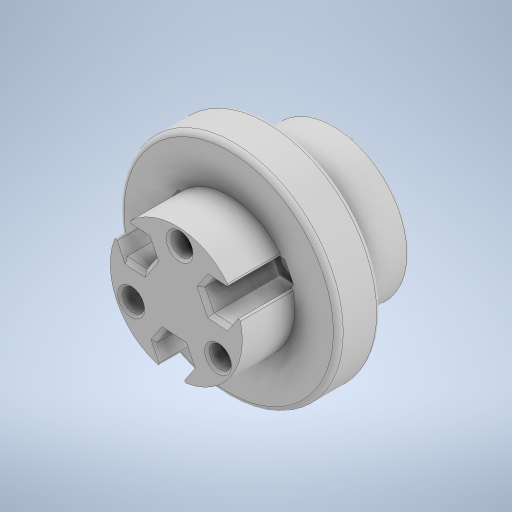
# Autodesk Inventor part: Os_lewa
Saved by Autodesk Inventor 2023 (Build 270158000, 158)
## iProperties
Created: 2023-01-20
Part Number: Os_lewa
Material: Generic
Document SubType Name: Modeling
Designer: Kamil
Density: 1 g/cm^3
Appearance: Default
Mass: 24.6075 g
Surface Area: 89.1781 cm^2
Volume: 24.6075 cm^3
Author: Kamil
Autodesk Inventor part; units mm, degrees
ref_plane "YZ Plane" through (0, 0, 0) normal (1, 0, 0) x (0, 1, 0)
ref_plane "XZ Plane" through (0, 0, 0) normal (0, 1, 0) x (-1, 0, 0)
sketch "Sketch1" plane through (0, 0, 0) normal (0, 0, 1) x (1, 0, 0)
  circle A0 centre (0, 0) radius 23.3333 projected
  arc A1 (-39.2843, 4.1223) -> (-36.4252, -2.8784) centre (-31.328, 3.2874) ccw projected
  arc A2 (-35.6202, -8.1415) -> (-36.4252, -2.8784) centre (-38.9739, -5.9614) ccw projected
  arc A3 (-35.6202, -8.1415) -> (-36.2558, -15.6768) centre (-28.9129, -12.5018) ccw projected
  arc A4 (-36.2558, -15.6768) -> (33.8969, -20.2792) centre (0, 0) ccw projected
  arc A5 (33.8969, -20.2792) -> (34.2512, -12.7254) centre (27.0317, -16.172) ccw projected
  arc A6 (35.737, -7.6127) -> (34.2512, -12.7254) centre (37.861, -11.0021) ccw projected
  arc A7 (35.737, -7.6127) -> (39.4862, -1.0454) centre (31.489, -0.8337) ccw projected
  arc A8 (39.4862, -1.0454) -> (-39.2843, 4.1223) centre (0, 0) ccw projected
  circle A9 centre (-9.1932, -4.5329) radius 2 projected
  circle A10 centre (9.1932, 4.5329) radius 2 projected
  circle A11 centre (-0.671, -10.228) radius 2 projected
  circle A12 centre (-8.5222, 5.6951) radius 2 projected
  circle A13 centre (0.671, 10.228) radius 2 projected
  circle A14 centre (8.5222, -5.6951) radius 2 projected
  circle A15 centre (0, 0) radius 13.4591 projected
  line L0 (-5.9382, 0.859) -> (-7.1311, 0.7284) projected
  arc A16 (-5.6118, -2.1232) -> (-5.9382, 0.859) centre (0, 0) ccw projected
  line L1 (-6.8047, -2.2538) -> (-5.6118, -2.1232) projected
  line L2 (-7.1311, 0.7284) -> (-6.8047, -2.2538) projected
  line L3 (23.3333, 0) -> (22.3333, 0)
  circle A17 centre (0, 0) radius 22.3333
  circle A18 centre (0, 0) radius 6
  circle A19 centre (16.7628, -26.571) radius 3.75 projected
  circle A20 centre (-29.1794, 11.6435) radius 3.75 projected
  circle A21 centre (2.0567, 31.3493) radius 3.75 projected
  circle A22 centre (-20.0905, -24.1532) radius 3.75 projected
  circle A23 centre (30.4505, 7.7314) radius 3.75 projected
  point P0 (0, 0)
  dimension "d0" = 1
  constraints: 2 coincident, 2 end point, 2 horizontal alignment, 1 horizontal, 6 other
  measures "d0" distance of L3.start L3.end
extrude "Extrusion1" add sketch "Sketch1" along normal blind 3.8 contours A15 | A18 L1 L2 L0 | A16 A18 | A17
sketch "Sketch2" plane through (0, 0, 0) normal (0, 0, -1) x (-1, 0, 0)
  circle A0 centre (0, 0) radius 15 projected
  circle A1 centre (0, 0) radius 22.3333 projected
  circle A2 centre (9.1932, -4.5329) radius 2 projected
  circle A3 centre (-9.1932, 4.5329) radius 2 projected
  circle A4 centre (0.671, -10.228) radius 2 projected
  circle A5 centre (8.5222, 5.6951) radius 2 projected
  circle A6 centre (-0.671, 10.228) radius 2 projected
  circle A7 centre (-8.5222, -5.6951) radius 2 projected
  point P0 (0, 0)
ref_plane "Work Plane1" through (-21.6708, -21.6708, -13) normal (0, 0, -1) x (0, 1, 0)
extrude "Extrusion2" add sketch "Sketch2" along normal up to surface (13 mm away) contours A0
sketch "Sketch3" plane through (0, 0, 3.8) normal (0, 0, 1) x (1, 0, 0)
  point P0 (0, 0)
sketch "Sketch4" plane through (0, 0, -13) normal (0, 0, -1) x (-1, 0, 0)
  circle A0 centre (0, 0) radius 15 projected
  circle A1 centre (-8.5222, -5.6951) radius 2 projected
  circle A2 centre (-0.671, 10.228) radius 2 projected
  circle A3 centre (8.5222, 5.6951) radius 2 projected
  circle A4 centre (0.671, -10.228) radius 2 projected
  circle A5 centre (-9.1932, 4.5329) radius 2 projected
  circle A6 centre (9.1932, -4.5329) radius 2 projected
  line L0 (0, 0) -> (9.1932, -4.5329)
  line L1 (9.1932, -4.5329) -> (12.3324, -6.0807)
  circle A7 centre (9.1932, -4.5329) radius 2 projected
  circle A8 centre (9.1932, -4.5329) radius 3.5
  circle A9 centre (8.5222, 5.6951) radius 3.5
  circle A10 centre (-0.671, 10.228) radius 3.5
  circle A11 centre (-9.1932, 4.5329) radius 3.5
  circle A12 centre (-8.5222, -5.6951) radius 3.5
  circle A13 centre (0.671, -10.228) radius 3.5
  point P0 (0, 0)
  point P1 (11.4322, 7.6398)
  point P2 (-0.9001, 13.7205)
  point P3 (-12.3324, 6.0807)
  point P4 (-11.4322, -7.6398)
  point P5 (0.9001, -13.7205)
  dimension "d5" = 3.5
  dimension "d8" = 360
  constraints: 4 end point, 1 coincident, 1 collinear, 37 other
  measures "d5" distance of L0.end L1.end
extrude "Extrusion3" cut sketch "Sketch4" against normal blind 5 contours A1 | A6 L1 L0 | A6 L0 A8 L1 | L0 L1 A6 | A6 L1 A8 L0 | A10 | A12
sketch "Sketch5" plane through (0, 0, 3.8) normal (0, 0, 1) x (1, 0, 0)
  circle A0 centre (0, 0) radius 22.3333 projected
  circle A1 centre (-9.1932, -4.5329) radius 2 projected
  circle A2 centre (9.1932, 4.5329) radius 2 projected
  circle A3 centre (-0.671, -10.228) radius 2 projected
  circle A4 centre (-8.5222, 5.6951) radius 2 projected
  circle A5 centre (0.671, 10.228) radius 2 projected
  circle A6 centre (8.5222, -5.6951) radius 2 projected
  line L0 (0, 0) -> (-0.671, -10.228)
  circle A7 centre (-0.671, -10.228) radius 2 projected
  line L1 (-0.671, -10.228) -> (-1.462, -22.2854)
  circle A8 centre (0, 0) radius 22.3333 projected
  line L2 (-0.671, -10.228) -> (-0.9001, -13.7205)
  line L3 (-3.0871, -13.8731) -> (-5.0083, -9.9765)
  line L4 (-5.0083, -9.9765) -> (-2.5944, -6.3644)
  line L5 (-2.5944, -6.3644) -> (1.7407, -6.6488)
  line L6 (1.7407, -6.6488) -> (3.662, -10.5454)
  line L7 (3.662, -10.5454) -> (1.2481, -14.1575)
  line L8 (1.2481, -14.1575) -> (-3.0871, -13.8731)
  line L9 (4.2145, -5.429) -> (6.6284, -1.8169)
  line L10 (6.1358, -9.3256) -> (4.2145, -5.429)
  line L11 (10.4709, -9.61) -> (6.1358, -9.3256)
  line L12 (12.8848, -5.9979) -> (10.4709, -9.61)
  line L13 (10.9635, -2.1013) -> (12.8848, -5.9979)
  line L14 (6.6284, -1.8169) -> (10.9635, -2.1013)
  line L15 (6.8089, 0.9353) -> (4.8877, 4.8319)
  line L16 (11.1441, 0.6509) -> (6.8089, 0.9353)
  line L17 (13.558, 4.2631) -> (11.1441, 0.6509)
  line L18 (11.6367, 8.1596) -> (13.558, 4.2631)
  line L19 (7.3016, 8.4441) -> (11.6367, 8.1596)
  line L20 (4.8877, 4.8319) -> (7.3016, 8.4441)
  line L21 (2.5944, 6.3644) -> (-1.7407, 6.6488)
  line L22 (5.0083, 9.9765) -> (2.5944, 6.3644)
  line L23 (3.0871, 13.8731) -> (5.0083, 9.9765)
  line L24 (-1.2481, 14.1575) -> (3.0871, 13.8731)
  line L25 (-3.662, 10.5454) -> (-1.2481, 14.1575)
  line L26 (-1.7407, 6.6488) -> (-3.662, 10.5454)
  line L27 (-4.2145, 5.429) -> (-6.6284, 1.8169)
  line L28 (-6.1358, 9.3256) -> (-4.2145, 5.429)
  line L29 (-10.4709, 9.61) -> (-6.1358, 9.3256)
  line L30 (-12.8848, 5.9979) -> (-10.4709, 9.61)
  line L31 (-10.9635, 2.1013) -> (-12.8848, 5.9979)
  line L32 (-6.6284, 1.8169) -> (-10.9635, 2.1013)
  line L33 (-6.8089, -0.9353) -> (-4.8877, -4.8319)
  line L34 (-11.1441, -0.6509) -> (-6.8089, -0.9353)
  line L35 (-13.558, -4.2631) -> (-11.1441, -0.6509)
  line L36 (-11.6367, -8.1596) -> (-13.558, -4.2631)
  line L37 (-7.3016, -8.4441) -> (-11.6367, -8.1596)
  line L38 (-4.8877, -4.8319) -> (-7.3016, -8.4441)
  point P0 (0, 0)
  point P1 (-0.6732, -10.261)
  point P2 (-0.9195, -14.0153)
  point P3 (11.6779, -7.8039)
  point P4 (12.5974, 6.2114)
  point P5 (0.9195, 14.0153)
  point P6 (-11.6779, 7.8039)
  point P7 (-12.5974, -6.2114)
  dimension "d13" = 3.5
  dimension "d16" = 360
  constraints: 78 end point, 2 point on line, 1 collinear, 1 midpoint, 94 other
  measures "d13" distance of L1.start L2.end
extrude "Extrusion4" add sketch "Sketch5" along normal blind 5 contours A0 | L9 L14 L13 L12 L11 L10 | L21 L26 L25 L24 L23 L22 | L33 L38 L37 L36 L35 L34
sketch "Sketch6" plane through (0, 0, 3.8) normal (0, 0, 1) x (1, 0, 0)
  line L0 (6.8089, 0.9353) -> (11.1441, 0.6509) projected
  line L1 (11.1441, 0.6509) -> (13.558, 4.2631) projected
  line L2 (13.558, 4.2631) -> (11.6367, 8.1596) projected
  line L3 (11.6367, 8.1596) -> (7.3016, 8.4441) projected
  line L4 (7.3016, 8.4441) -> (4.8877, 4.8319) projected
  line L5 (4.8877, 4.8319) -> (6.8089, 0.9353) projected
  circle A0 centre (9.1932, 4.5329) radius 2 projected
  circle A1 centre (0, 0) radius 22.3333 projected
  circle A2 centre (8.5222, -5.6951) radius 2 projected
  circle A3 centre (0.671, 10.228) radius 2 projected
  circle A4 centre (-9.1932, -4.5329) radius 2 projected
  line L6 (1.2481, -14.1575) -> (-3.0871, -13.8731) projected
  line L7 (-3.0871, -13.8731) -> (-5.0083, -9.9765) projected
  line L8 (-5.0083, -9.9765) -> (-2.5944, -6.3644) projected
  line L9 (-2.5944, -6.3644) -> (1.7407, -6.6488) projected
  line L10 (1.7407, -6.6488) -> (3.662, -10.5454) projected
  line L11 (3.662, -10.5454) -> (1.2481, -14.1575) projected
  line L12 (-4.2145, 5.429) -> (-6.6284, 1.8169) projected
  line L13 (-6.6284, 1.8169) -> (-10.9635, 2.1013) projected
  line L14 (-10.9635, 2.1013) -> (-12.8848, 5.9979) projected
  line L15 (-12.8848, 5.9979) -> (-10.4709, 9.61) projected
  line L16 (-10.4709, 9.61) -> (-6.1358, 9.3256) projected
  line L17 (-6.1358, 9.3256) -> (-4.2145, 5.429) projected
  line L18 (6.8089, 0.9353) -> (4.8877, 4.8319) projected
  line L19 (4.8877, 4.8319) -> (7.3016, 8.4441) projected
  line L20 (7.3016, 8.4441) -> (11.6367, 8.1596) projected
  line L21 (11.6367, 8.1596) -> (13.558, 4.2631) projected
  line L22 (13.558, 4.2631) -> (11.1441, 0.6509) projected
  line L23 (11.1441, 0.6509) -> (6.8089, 0.9353) projected
  circle A5 centre (-0.671, -10.228) radius 2 projected
  circle A6 centre (-8.5222, 5.6951) radius 2 projected
  point P0 (0, 0)
extrude "Extrusion5" add sketch "Sketch6" along normal blind 1.5 contours L5 L4 L3 L2 L1 L0 | L6 L7 L8 L9 L10 L11 | L12 L13 L14 L15 L16 L17
sketch "Sketch7" plane through (0, 0, 8.8) normal (0, 0, 1) x (1, 0, 0)
  circle A0 centre (8.5222, -5.6951) radius 2 projected
  circle A1 centre (9.1932, 4.5329) radius 2 projected
  circle A2 centre (-0.671, -10.228) radius 2 projected
  circle A3 centre (0.671, 10.228) radius 2 projected
  circle A4 centre (-9.1932, -4.5329) radius 2 projected
  arc A5 (5.9995, 0.0758) -> (5.2863, -2.8382) centre (0, 0) ccw projected
  line L0 (7.1651, -0.2095) -> (5.9995, 0.0758) projected
  line L1 (6.4519, -3.1235) -> (7.1651, -0.2095) projected
  line L2 (5.2863, -2.8382) -> (6.4519, -3.1235) projected
  circle A6 centre (-8.5222, 5.6951) radius 2 projected
  circle A7 centre (0, 0) radius 13.4542 projected
  circle A8 centre (0, 0) radius 6
  circle A9 centre (0, 0) radius 22.3333 projected
  circle A10 centre (8.5222, -5.6951) radius 2 projected
  circle A11 centre (0.671, 10.228) radius 2 projected
  circle A12 centre (-9.1932, -4.5329) radius 2 projected
  line L3 (1.2481, -14.1575) -> (-3.0871, -13.8731) projected
  line L4 (-3.0871, -13.8731) -> (-5.0083, -9.9765) projected
  line L5 (-5.0083, -9.9765) -> (-2.5944, -6.3644) projected
  line L6 (-2.5944, -6.3644) -> (1.7407, -6.6488) projected
  line L7 (1.7407, -6.6488) -> (3.662, -10.5454) projected
  line L8 (3.662, -10.5454) -> (1.2481, -14.1575) projected
  line L9 (-4.2145, 5.429) -> (-6.6284, 1.8169) projected
  line L10 (-6.6284, 1.8169) -> (-10.9635, 2.1013) projected
  line L11 (-10.9635, 2.1013) -> (-12.8848, 5.9979) projected
  line L12 (-12.8848, 5.9979) -> (-10.4709, 9.61) projected
  line L13 (-10.4709, 9.61) -> (-6.1358, 9.3256) projected
  line L14 (-6.1358, 9.3256) -> (-4.2145, 5.429) projected
  line L15 (6.8089, 0.9353) -> (4.8877, 4.8319) projected
  line L16 (4.8877, 4.8319) -> (7.3016, 8.4441) projected
  line L17 (7.3016, 8.4441) -> (11.6367, 8.1596) projected
  line L18 (11.6367, 8.1596) -> (13.558, 4.2631) projected
  line L19 (13.558, 4.2631) -> (11.1441, 0.6509) projected
  line L20 (11.1441, 0.6509) -> (6.8089, 0.9353) projected
  point P0 (0, 0)
  point P1 (1.7989, -13.3334)
  point P2 (13.0072, 3.4389)
  point P3 (10.6476, 8.2245)
  point P4 (-9.4818, 9.5451)
  point P5 (-12.4465, 5.1088)
  point P6 (-3.5254, -12.9841)
  constraints: 1 coincident, 3 other
extrude "Extrusion6" add sketch "Sketch7" along normal blind 5.2 contours L0 L1 L2 A8 | A7 L8 L7 L6 L5 L4 L11 L10 L9 L14 L13 L17 L16 L15 L20 L19
sketch "Sketch8" plane through (-9.1932, -4.5329, -8) normal (0, 0, -1) x (-1, 0, 0)
  circle A0 centre (0, 0) radius 2 projected
  circle A1 centre (0, 0) radius 3.5 projected
  circle A2 centre (-9.8642, 14.7609) radius 3.5 projected
  circle A3 centre (-17.7154, -1.1622) radius 3.5 projected
  circle A4 centre (0, 0) radius 3.5 projected
  circle A5 centre (-9.1932, 4.5329) radius 15 projected
  circle A6 centre (-0.671, 10.228) radius 2 projected
  circle A7 centre (-8.5222, -5.6951) radius 2 projected
  circle A8 centre (-18.3864, 9.0658) radius 2 projected
  line L0 (0, 0) -> (-18.3864, 9.0658)
  line L1 (-17.7154, -1.1622) -> (-0.671, 10.228)
  line L2 (-8.5222, -5.6951) -> (-9.8642, 14.7609)
  line L3 (0, 0) -> (3.1391, -1.5478)
  line L4 (2.2455, -3.3602) -> (-1.7873, -3.6248)
  line L5 (-1.7873, -3.6248) -> (-4.0328, -0.2646)
  line L6 (-4.0328, -0.2646) -> (-2.2455, 3.3602)
  line L7 (-2.2455, 3.3602) -> (1.7873, 3.6248)
  line L8 (1.7873, 3.6248) -> (4.0328, 0.2646)
  line L9 (4.0328, 0.2646) -> (2.2455, -3.3602)
  line L10 (3.3618, 10.4926) -> (1.5745, 6.8678)
  line L11 (1.5745, 6.8678) -> (-2.4583, 6.6032)
  line L12 (-2.4583, 6.6032) -> (-4.7038, 9.9634)
  line L13 (-4.7038, 9.9634) -> (-2.9165, 13.5882)
  line L14 (-2.9165, 13.5882) -> (1.1163, 13.8528)
  line L15 (1.1163, 13.8528) -> (3.3618, 10.4926)
  line L16 (-8.077, 18.3857) -> (-5.8315, 15.0255)
  line L17 (-5.8315, 15.0255) -> (-7.6187, 11.4007)
  line L18 (-7.6187, 11.4007) -> (-11.6515, 11.1361)
  line L19 (-11.6515, 11.1361) -> (-13.897, 14.4963)
  line L20 (-13.897, 14.4963) -> (-12.1097, 18.1211)
  line L21 (-12.1097, 18.1211) -> (-8.077, 18.3857)
  line L22 (-20.632, 12.426) -> (-16.5992, 12.6906)
  line L23 (-16.5992, 12.6906) -> (-14.3537, 9.3304)
  line L24 (-14.3537, 9.3304) -> (-16.1409, 5.7056)
  line L25 (-16.1409, 5.7056) -> (-20.1737, 5.441)
  line L26 (-20.1737, 5.441) -> (-22.4192, 8.8012)
  line L27 (-22.4192, 8.8012) -> (-20.632, 12.426)
  line L28 (-21.7482, -1.4268) -> (-19.961, 2.198)
  line L29 (-19.961, 2.198) -> (-15.9282, 2.4626)
  line L30 (-15.9282, 2.4626) -> (-13.6827, -0.8977)
  line L31 (-13.6827, -0.8977) -> (-15.4699, -4.5224)
  line L32 (-15.4699, -4.5224) -> (-19.5027, -4.787)
  line L33 (-19.5027, -4.787) -> (-21.7482, -1.4268)
  line L34 (-10.3095, -9.3199) -> (-12.555, -5.9597)
  line L35 (-12.555, -5.9597) -> (-10.7677, -2.3349)
  line L36 (-10.7677, -2.3349) -> (-6.7349, -2.0703)
  line L37 (-6.7349, -2.0703) -> (-4.4894, -5.4305)
  line L38 (-4.4894, -5.4305) -> (-6.2767, -9.0553)
  line L39 (-6.2767, -9.0553) -> (-10.3095, -9.3199)
  point P0 (-9.1932, 4.5329)
  point P1 (2.239, 12.1727)
  point P2 (-10.0934, 18.2534)
  point P3 (-21.5256, 10.6136)
  point P4 (-20.6255, -3.1069)
  point P5 (-8.2931, -9.1876)
  dimension "d24" = 3.5
  dimension "d27" = 360
  constraints: 80 end point, 1 coincident, 1 collinear, 1 midpoint, 92 other
  measures "d24" distance of L0.start L3.end
extrude "Extrusion7" cut sketch "Sketch8" along normal blind 10 contours A0 L3 L0 | A0 L0 A1 L3 | L0 L3 A0 | A0 L3 A1 L0 | L6 L7 A1 | A1 L5 L6 | L9 L4 A1 | A1 L8 L9 | L7 L8 A1 | A1 L4 L5 | A2 | A2 L16 L17 | A2 L21 L16 | L17 L18 A2 | A2 L20 L21 | L18 L19 A2 | A2 L19 L20 | A3 | A3 L30 L31 | A3 L29 L30 | L31 L32 A3 | A3 L28 L29 | L32 L33 A3 | A3 L33 L28
sketch "Sketch9" plane through (0, 0, 8.8) normal (0, 0, 1) x (1, 0, 0)
  circle A0 centre (0, 0) radius 6 projected
  point P0 (0, 0)
extrude "Extrusion8" add sketch "Sketch9" along normal up to surface (5.2 mm away)
sketch "Sketch10" plane through (0, 0, 14) normal (0, 0, 1) x (1, 0, 0)
  line L0 (3.662, -10.5454) -> (1.7989, -13.3334) projected
  arc A0 (1.7989, -13.3334) -> (13.0072, 3.4389) centre (0, 0) ccw projected
  line L1 (13.0072, 3.4389) -> (11.1441, 0.6509) projected
  line L2 (11.1441, 0.6509) -> (6.8089, 0.9353) projected
  line L3 (6.8089, 0.9353) -> (4.8877, 4.8319) projected
  line L4 (4.8877, 4.8319) -> (7.3016, 8.4441) projected
  line L5 (7.3016, 8.4441) -> (10.6476, 8.2245) projected
  arc A1 (10.6476, 8.2245) -> (-9.4818, 9.5451) centre (0, 0) ccw projected
  line L6 (-9.4818, 9.5451) -> (-6.1358, 9.3256) projected
  line L7 (-6.1358, 9.3256) -> (-4.2145, 5.429) projected
  line L8 (-4.2145, 5.429) -> (-6.6284, 1.8169) projected
  line L9 (-6.6284, 1.8169) -> (-10.9635, 2.1013) projected
  line L10 (-10.9635, 2.1013) -> (-12.4465, 5.1088) projected
  arc A2 (-12.4465, 5.1088) -> (-3.5254, -12.9841) centre (0, 0) ccw projected
  line L11 (-3.5254, -12.9841) -> (-5.0083, -9.9765) projected
  line L12 (-5.0083, -9.9765) -> (-2.5944, -6.3644) projected
  line L13 (-2.5944, -6.3644) -> (1.7407, -6.6488) projected
  line L14 (1.7407, -6.6488) -> (3.662, -10.5454) projected
  circle A3 centre (8.5222, -5.6951) radius 2 projected
  circle A4 centre (0.671, 10.228) radius 2 projected
  circle A5 centre (-9.1932, -4.5329) radius 2 projected
  point P0 (0, 0)
extrude "Extrusion9" add sketch "Sketch10" along normal blind 5.5
sketch "Sketch11" plane through (0, 0, 19.5) normal (0, 0, 1) x (1, 0, 0)
  line L0 (-5.0083, -9.9765) -> (-2.5944, -6.3644) projected
  line L1 (-2.5944, -6.3644) -> (1.7407, -6.6488) projected
  line L2 (1.7407, -6.6488) -> (3.662, -10.5454) projected
  line L3 (11.1441, 0.6509) -> (6.8089, 0.9353) projected
  line L4 (6.8089, 0.9353) -> (4.8877, 4.8319) projected
  line L5 (4.8877, 4.8319) -> (7.3016, 8.4441) projected
  line L6 (-6.1358, 9.3256) -> (-4.2145, 5.429) projected
  line L7 (-4.2145, 5.429) -> (-6.6284, 1.8169) projected
  line L8 (-6.6284, 1.8169) -> (-10.9635, 2.1013) projected
  circle A0 centre (-9.1932, -4.5329) radius 2 projected
  circle A1 centre (0.671, 10.228) radius 2 projected
  circle A2 centre (8.5222, -5.6951) radius 2 projected
  circle A3 centre (-8.5222, 5.6951) radius 2 projected
  circle A4 centre (-0.671, -10.228) radius 2 projected
  circle A5 centre (9.1932, 4.5329) radius 2 projected
  circle A6 centre (-8.5222, 5.6951) radius 2 projected
  circle A7 centre (-8.5222, 5.6951) radius 2.25
  circle A8 centre (0.671, 10.228) radius 2 projected
  circle A9 centre (0.671, 10.228) radius 2.25
  circle A10 centre (9.1932, 4.5329) radius 2.25
  circle A11 centre (-0.671, -10.228) radius 2 projected
  circle A12 centre (-0.671, -10.228) radius 2.25
  circle A13 centre (-9.1932, -4.5329) radius 2.25
  circle A14 centre (8.5222, -5.6951) radius 2.25
  line L9 (-3.5254, -12.9841) -> (-5.0083, -9.9765) projected
  line L10 (3.662, -10.5454) -> (1.7989, -13.3334) projected
  line L11 (13.0072, 3.4389) -> (11.1441, 0.6509) projected
  line L12 (7.3016, 8.4441) -> (10.6476, 8.2245) projected
  line L13 (-9.4818, 9.5451) -> (-6.1358, 9.3256) projected
  line L14 (-10.9635, 2.1013) -> (-12.4465, 5.1088) projected
  arc A15 (1.7989, -13.3334) -> (13.0072, 3.4389) centre (0, 0) ccw projected
  arc A16 (10.6476, 8.2245) -> (-9.4818, 9.5451) centre (0, 0) ccw projected
  arc A17 (-12.4465, 5.1088) -> (-3.5254, -12.9841) centre (0, 0) ccw projected
  point P0 (0, 0)
  dimension "d37" = 4.5
  dimension "d38" = 4.5
  dimension "d39" = 4.5
  dimension "d40" = 4.5
  dimension "d41" = 4.5
  dimension "d42" = 4.5
  constraints: 6 centre point, 6 coincident
  measures "d37" diameter of A7
  measures "d38" diameter of A9
  measures "d39" diameter of A10
  measures "d40" diameter of A12
  measures "d41" diameter of A13
  measures "d42" diameter of A14
extrude "Extrusion10" cut sketch "Sketch11" against normal through all contours A0 | A1 | A2 | A3 | A4 | A5 | A7 | A9 | A10 | A12 | A13 | A14
sketch "Sketch13" plane through (0, 0, -8) normal (0, 0, -1) x (-1, 0, 0)
  circle A0 centre (-8.5222, -5.6951) radius 2.25 projected
  line L0 (-6.7349, -2.0703) -> (-10.7677, -2.3349) projected
  line L1 (-10.7677, -2.3349) -> (-12.555, -5.9597) projected
  line L2 (-12.555, -5.9597) -> (-10.3095, -9.3199) projected
  line L3 (-10.3095, -9.3199) -> (-6.2767, -9.0553) projected
  line L4 (-6.2767, -9.0553) -> (-4.4894, -5.4305) projected
  line L5 (-4.4894, -5.4305) -> (-6.7349, -2.0703) projected
  circle A1 centre (9.1932, -4.5329) radius 2.25 projected
  line L6 (13.226, -4.2683) -> (10.9805, -0.9081) projected
  line L7 (10.9805, -0.9081) -> (6.9477, -1.1727) projected
  line L8 (6.9477, -1.1727) -> (5.1604, -4.7975) projected
  line L9 (5.1604, -4.7975) -> (7.406, -8.1577) projected
  line L10 (7.406, -8.1577) -> (11.4387, -7.8931) projected
  line L11 (11.4387, -7.8931) -> (13.226, -4.2683) projected
  circle A2 centre (-0.671, 10.228) radius 2.25 projected
  line L12 (1.5745, 6.8678) -> (3.3618, 10.4926) projected
  line L13 (3.3618, 10.4926) -> (1.1163, 13.8528) projected
  line L14 (1.1163, 13.8528) -> (-2.9165, 13.5882) projected
  line L15 (-2.9165, 13.5882) -> (-4.7038, 9.9634) projected
  line L16 (-4.7038, 9.9634) -> (-2.4583, 6.6032) projected
  line L17 (-2.4583, 6.6032) -> (1.5745, 6.8678) projected
  point P0 (0, 0)
extrude "Extrusion12" cut sketch "Sketch13" against normal blind 3
sketch "Szkic14" plane through (0, 0, 5.3) normal (0, 0, 1) x (1, 0, 0)
  circle A0 centre (-8.5222, 5.6951) radius 2.25 projected
  line L0 (-10.4709, 9.61) -> (-6.1358, 9.3256) projected
  line L1 (-12.8848, 5.9979) -> (-10.4709, 9.61) projected
  line L2 (-10.9635, 2.1013) -> (-12.8848, 5.9979) projected
  line L3 (-6.6284, 1.8169) -> (-10.9635, 2.1013) projected
  line L4 (-4.2145, 5.429) -> (-6.6284, 1.8169) projected
  line L5 (-6.1358, 9.3256) -> (-4.2145, 5.429) projected
  circle A1 centre (-0.671, -10.228) radius 2.25 projected
  line L6 (1.7407, -6.6488) -> (3.662, -10.5454) projected
  line L7 (-2.5944, -6.3644) -> (1.7407, -6.6488) projected
  line L8 (-5.0083, -9.9765) -> (-2.5944, -6.3644) projected
  line L9 (-3.0871, -13.8731) -> (-5.0083, -9.9765) projected
  line L10 (1.2481, -14.1575) -> (-3.0871, -13.8731) projected
  line L11 (3.662, -10.5454) -> (1.2481, -14.1575) projected
  circle A2 centre (9.1932, 4.5329) radius 2.25 projected
  line L12 (11.1441, 0.6509) -> (6.8089, 0.9353) projected
  line L13 (13.558, 4.2631) -> (11.1441, 0.6509) projected
  line L14 (11.6367, 8.1596) -> (13.558, 4.2631) projected
  line L15 (7.3016, 8.4441) -> (11.6367, 8.1596) projected
  line L16 (4.8877, 4.8319) -> (7.3016, 8.4441) projected
  line L17 (6.8089, 0.9353) -> (4.8877, 4.8319) projected
  line L18 (-8.5222, 5.6951) -> (-8.2931, 9.1876)
  line L19 (-6.2767, 9.0553) -> (-4.4894, 5.4305)
  line L20 (-4.4894, 5.4305) -> (-6.7349, 2.0703)
  line L21 (-6.7349, 2.0703) -> (-10.7677, 2.3349)
  line L22 (-10.7677, 2.3349) -> (-12.555, 5.9597)
  line L23 (-12.555, 5.9597) -> (-10.3095, 9.3199)
  line L24 (-10.3095, 9.3199) -> (-6.2767, 9.0553)
  line L25 (-9.4818, 9.5451) -> (-6.1358, 9.3256) projected
  circle A3 centre (-9.1932, -4.5329) radius 2.25 projected
  circle A4 centre (0.671, 10.228) radius 2.25 projected
  circle A5 centre (8.5222, -5.6951) radius 2.25 projected
  arc A6 (1.7989, -13.3334) -> (13.0072, 3.4389) centre (0, 0) ccw projected
  line L26 (13.0072, 3.4389) -> (11.1441, 0.6509) projected
  line L27 (11.1441, 0.6509) -> (6.8089, 0.9353) projected
  line L28 (6.8089, 0.9353) -> (4.8877, 4.8319) projected
  line L29 (4.8877, 4.8319) -> (7.3016, 8.4441) projected
  line L30 (7.3016, 8.4441) -> (10.6476, 8.2245) projected
  arc A7 (10.6476, 8.2245) -> (-9.4818, 9.5451) centre (0, 0) ccw projected
  line L31 (-9.4818, 9.5451) -> (-6.1358, 9.3256) projected
  line L32 (-6.1358, 9.3256) -> (-4.2145, 5.429) projected
  line L33 (-4.2145, 5.429) -> (-6.6284, 1.8169) projected
  line L34 (-6.6284, 1.8169) -> (-10.9635, 2.1013) projected
  line L35 (-10.9635, 2.1013) -> (-12.4465, 5.1088) projected
  arc A8 (-12.4465, 5.1088) -> (-3.5254, -12.9841) centre (0, 0) ccw projected
  line L36 (-3.5254, -12.9841) -> (-5.0083, -9.9765) projected
  line L37 (-5.0083, -9.9765) -> (-2.5944, -6.3644) projected
  line L38 (-2.5944, -6.3644) -> (1.7407, -6.6488) projected
  line L39 (1.7407, -6.6488) -> (3.662, -10.5454) projected
  line L40 (3.662, -10.5454) -> (1.7989, -13.3334) projected
  arc A9 (10.6476, 8.2245) -> (-9.4818, 9.5451) centre (0, 0) ccw projected
  line L41 (10.6476, 8.2245) -> (11.6367, 8.1596) projected
  line L42 (11.6367, 8.1596) -> (13.558, 4.2631) projected
  line L43 (13.558, 4.2631) -> (13.0072, 3.4389) projected
  arc A10 (1.7989, -13.3334) -> (13.0072, 3.4389) centre (0, 0) ccw projected
  line L44 (1.7989, -13.3334) -> (1.2481, -14.1575) projected
  line L45 (1.2481, -14.1575) -> (-3.0871, -13.8731) projected
  line L46 (-3.0871, -13.8731) -> (-3.5254, -12.9841) projected
  arc A11 (-12.4465, 5.1088) -> (-3.5254, -12.9841) centre (0, 0) ccw projected
  line L47 (-12.4465, 5.1088) -> (-12.8848, 5.9979) projected
  line L48 (-12.8848, 5.9979) -> (-10.4709, 9.61) projected
  line L49 (-10.4709, 9.61) -> (-9.4818, 9.5451) projected
  circle A12 centre (0, 0) radius 22.3333 projected
  line L50 (-10.9805, -0.9081) -> (-6.9477, -1.1727)
  line L51 (-13.226, -4.2683) -> (-10.9805, -0.9081)
  line L52 (-11.4387, -7.8931) -> (-13.226, -4.2683)
  line L53 (-7.406, -8.1577) -> (-11.4387, -7.8931)
  line L54 (-6.9477, -1.1727) -> (-5.1604, -4.7975)
  line L55 (-5.1604, -4.7975) -> (-7.406, -8.1577)
  line L56 (-4.7038, -9.9634) -> (-2.4583, -6.6032)
  line L57 (-2.9165, -13.5882) -> (-4.7038, -9.9634)
  line L58 (1.1163, -13.8528) -> (-2.9165, -13.5882)
  line L59 (3.3618, -10.4926) -> (1.1163, -13.8528)
  line L60 (-2.4583, -6.6032) -> (1.5745, -6.8678)
  line L61 (1.5745, -6.8678) -> (3.3618, -10.4926)
  line L62 (6.2767, -9.0553) -> (4.4894, -5.4305)
  line L63 (10.3095, -9.3199) -> (6.2767, -9.0553)
  line L64 (12.555, -5.9597) -> (10.3095, -9.3199)
  line L65 (10.7677, -2.3349) -> (12.555, -5.9597)
  line L66 (4.4894, -5.4305) -> (6.7349, -2.0703)
  line L67 (6.7349, -2.0703) -> (10.7677, -2.3349)
  line L68 (10.9805, 0.9081) -> (6.9477, 1.1727)
  line L69 (13.226, 4.2683) -> (10.9805, 0.9081)
  line L70 (11.4387, 7.8931) -> (13.226, 4.2683)
  line L71 (7.406, 8.1577) -> (11.4387, 7.8931)
  line L72 (6.9477, 1.1727) -> (5.1604, 4.7975)
  line L73 (5.1604, 4.7975) -> (7.406, 8.1577)
  line L74 (4.7038, 9.9634) -> (2.4583, 6.6032)
  line L75 (2.9165, 13.5882) -> (4.7038, 9.9634)
  line L76 (-1.1163, 13.8528) -> (2.9165, 13.5882)
  line L77 (-3.3618, 10.4926) -> (-1.1163, 13.8528)
  line L78 (2.4583, 6.6032) -> (-1.5745, 6.8678)
  line L79 (-1.5745, 6.8678) -> (-3.3618, 10.4926)
  point P0 (0, 0)
  point P1 (-12.1032, -2.5882)
  point P2 (-3.8102, -11.7758)
  point P3 (8.2931, -9.1876)
  point P4 (12.1032, 2.5882)
  point P5 (3.8102, 11.7758)
  dimension "d49" = 3.5
  dimension "d52" = 360
  constraints: 74 end point, 2 perpendicular, 1 coincident, 1 midpoint, 92 other
  measures "d49" distance of L18.start L18.end
extrude "Wyciągnięcie proste13" add sketch "Szkic14" along normal up to surface (14.2 mm away) contours L0 L5 L4 L3 L2 L1 | L15 L14 L13 L12 L17 L16 | L9 L8 L7 L6 L11 L10
sketch "Szkic15" plane through (0, 0, 19.5) normal (0, 0, 1) x (1, 0, 0)
  line L0 (10.9805, 0.9081) -> (13.226, 4.2683) projected
  line L1 (6.9477, 1.1727) -> (10.9805, 0.9081) projected
  line L2 (5.1604, 4.7975) -> (6.9477, 1.1727) projected
  line L3 (7.406, 8.1577) -> (5.1604, 4.7975) projected
  line L4 (11.4387, 7.8931) -> (7.406, 8.1577) projected
  line L5 (13.226, 4.2683) -> (11.4387, 7.8931) projected
  line L6 (-12.555, 5.9597) -> (-10.7677, 2.3349) projected
  line L7 (-10.3095, 9.3199) -> (-12.555, 5.9597) projected
  line L8 (-6.2767, 9.0553) -> (-10.3095, 9.3199) projected
  line L9 (-4.4894, 5.4305) -> (-6.2767, 9.0553) projected
  line L10 (-6.7349, 2.0703) -> (-4.4894, 5.4305) projected
  line L11 (-10.7677, 2.3349) -> (-6.7349, 2.0703) projected
  line L12 (-4.7038, -9.9634) -> (-2.9165, -13.5882) projected
  line L13 (-2.4583, -6.6032) -> (-4.7038, -9.9634) projected
  line L14 (1.5745, -6.8678) -> (-2.4583, -6.6032) projected
  line L15 (3.3618, -10.4926) -> (1.5745, -6.8678) projected
  line L16 (1.1163, -13.8528) -> (3.3618, -10.4926) projected
  line L17 (-2.9165, -13.5882) -> (1.1163, -13.8528) projected
  circle A0 centre (-9.1932, -4.5329) radius 2.25 projected
  circle A1 centre (0.671, 10.228) radius 2.25 projected
  circle A2 centre (8.5222, -5.6951) radius 2.25 projected
  line L18 (-3.0871, -13.8731) -> (-3.5254, -12.9841) projected
  line L19 (1.2481, -14.1575) -> (-3.0871, -13.8731) projected
  line L20 (1.7989, -13.3334) -> (1.2481, -14.1575) projected
  arc A3 (1.7989, -13.3334) -> (13.0072, 3.4389) centre (0, 0) ccw projected
  line L21 (13.558, 4.2631) -> (13.0072, 3.4389) projected
  line L22 (11.6367, 8.1596) -> (13.558, 4.2631) projected
  line L23 (10.6476, 8.2245) -> (11.6367, 8.1596) projected
  arc A4 (10.6476, 8.2245) -> (-9.4818, 9.5451) centre (0, 0) ccw projected
  line L24 (-10.4709, 9.61) -> (-9.4818, 9.5451) projected
  line L25 (-12.8848, 5.9979) -> (-10.4709, 9.61) projected
  line L26 (-12.4465, 5.1088) -> (-12.8848, 5.9979) projected
  arc A5 (-12.4465, 5.1088) -> (-3.5254, -12.9841) centre (0, 0) ccw projected
  circle A6 centre (0, 0) radius 13.4542
  point P0 (0, 0)
  point P1 (-9.7391, 9.2825)
  point P2 (-9.4818, 9.5451)
  point P3 (-12.3022, 5.447)
  point P4 (-3.1693, -13.0755)
  point P5 (1.4339, -13.3775)
  point P6 (12.9084, 3.7931)
  point P7 (13.0072, 3.4389)
  point P8 (10.8684, 7.9305)
  constraints: 1 centre point, 1 coincident, 1 concentric
extrude "Wyciągnięcie proste14" cut sketch "Szkic15" against normal up to surface (10.7 mm away) contours L0 L5 L4 A6 L23 L22 L21 | L20 L19 L18 A6 L12 L17 L16 | A6 L8 L7 L6 L26 L25 L24
fillet "Zaokrąglenie3" radius 1 2 edges at (-22.3333, 0, 0) (-22.3333, 0, 8.8)
fillet "Zaokrąglenie4" radius 0.3 6 edges at (12.9084, 3.7931, 14.15) (10.8684, 7.9305, 14.15) (1.4339, -13.3775, 14.15) (-3.1693, -13.0755, 14.15) (-12.3022, 5.447, 14.15) (-9.7391, 9.2825, 14.15)
chamfer "Faza1" distance 0.5 angle 45 6 edges at (-1.579, 10.228, 19.5) (6.2722, -5.6951, 19.5) (-11.4432, -4.5329, 19.5) (-10.7722, 5.6951, -13) (6.9432, 4.5329, -13) (-2.921, -10.228, -13)
chamfer "Faza2" distance 0.8 angle 45 27 edges at (-5.3831, 7.2429, 19.5) (-5.6122, 3.7504, 19.5) (-8.7513, 2.2026, 19.5) (-3.581, -8.2833, 19.5) (-0.4419, -6.7355, 19.5) (2.4681, -8.6802, 19.5) (6.2832, 6.4776, 19.5) (6.0541, 2.9851, 19.5) (8.9641, 1.0404, 19.5) (-6.2832, -6.4776, -13) (-9.4223, -8.0254, -13) (-12.3324, -6.0807, -13) (-12.1032, -2.5882, -13) (-8.9641, -1.0404, -13) (-6.0541, -2.9851, -13) (0.4419, 6.7355, -13) (-2.4681, 8.6802, -13) (-2.239, 12.1727, -13) (0.9001, 13.7205, -13) (3.8102, 11.7758, -13) (3.581, 8.2833, -13) (5.6122, -3.7504, -13) (5.3831, -7.2429, -13) (8.2931, -9.1876, -13) (11.4322, -7.6398, -13) (11.6614, -4.1473, -13) (8.7513, -2.2026, -13)
fillet "Zaokrąglenie5" radius 0.5 1 edges at (15, 0, -13)
body "Solid1"
